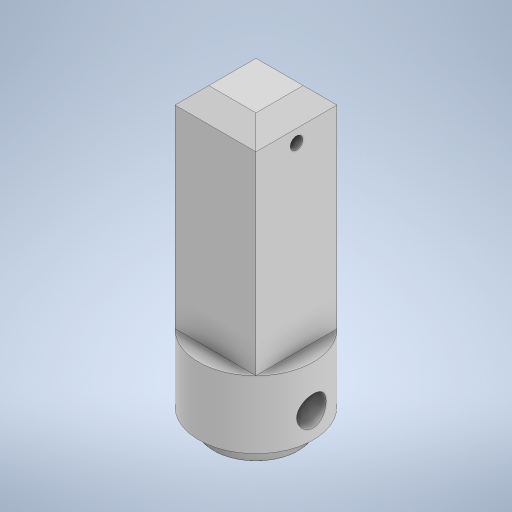
# Autodesk Inventor part: wheel-lockV2
Saved by Autodesk Inventor 2024.2 (Build 282272000, 272)
## iProperties
Created: 2024-04-01
Part Number: wheel-lockV2
Material: Generic
Document SubType Name: Modeling
Designer: Robin
Density: 1 g/cm^3
Appearance: Default
Author: Robin
Autodesk Inventor part; units mm, degrees
ref_plane "YZ Plane" through (0, 0, 0) normal (1, 0, 0) x (0, 1, 0)
ref_plane "XZ Plane" through (0, 0, 0) normal (0, 1, 0) x (-1, 0, 0)
ref_plane "XY Plane" through (0, 0, 0) normal (0, 0, 1) x (1, 0, 0)
sketch "Sketch1" plane through (0, 0, 0) normal (0, 1, 0) x (-1, 0, 0)
  line L0 (4.8, 4.8) -> (-4.8, 4.8)
  line L1 (-4.8, 4.8) -> (-4.8, -4.8)
  line L2 (-4.8, -4.8) -> (4.8, -4.8)
  line L3 (4.8, -4.8) -> (4.8, 4.8)
  point P0 (0, 0)
  point P1 (4.8, 0)
  point P2 (0, -4.8)
  dimension "d0" = 9.6
  dimension "d1" = 9.6
  constraints: 8 end point, 2 midpoint, 2 parallel, 1 horizontal, 1 horizontal alignment, 1 perpendicular, 1 vertical alignment
  measures "d0" distance of L2.end L0.start
  measures "d1" distance of L1.end L2.end
extrude "Extrusion1" add sketch "Sketch1" along normal blind 35
sketch "Sketch5" plane through (0, 0, 0) normal (0, -1, 0) x (1, 0, 0)
  circle A0 centre (0, 0) radius 2.1
  line L0 (4.8, 4.8) -> (4.8, -4.8) projected
  line L1 (-4.8, 4.8) -> (4.8, 4.8) projected
  line L2 (4.8, -4.8) -> (-4.8, -4.8) projected
  line L3 (4.8, 4.8) -> (-4.8, 4.8)
  line L4 (-4.8, 4.8) -> (-4.8, -4.8)
  line L5 (-4.8, -4.8) -> (4.8, -4.8)
  line L6 (4.8, -4.8) -> (4.8, 4.8)
  circle A1 centre (0, 0) radius 6.7882
  point P0 (-4.8, 4.8)
  point P1 (-4.8, 4.8)
  point P2 (-4.8, 4.8)
  dimension "d14" = 4.2
  constraints: 8 end point, 2 coincident, 2 parallel, 1 centre point, 1 horizontal, 1 perpendicular, 3 other
  measures "d14" diameter of A0
extrude "Extrusion5" add sketch "Sketch5" against normal blind 10 contours A1 L0 | L1 A1 | A1 L2 | L4 A1
sketch "Sketch6" plane through (4.8, 35, 4.8) normal (1, 0, 0) x (0, 0, -1)
  line L0 (0, 0) -> (9.6, 0) projected
  point P0 (4.8, -35)
  point P1 (4.8, -3.5)
  point P2 (4.8, 0)
  dimension "d18" = 3.5
  constraints: 1 midpoint, 1 vertical alignment
  measures "d18" distance from line of L0 point (4.8, -3.5)
hole "Hole1" at (4.8, 31.5, 0) direction (-1, 0, 0) diameter 1.5 end through all
sketch "Sketch9" plane through (4.8, 35, 4.8) normal (1, 0, 0) x (0, 0, -1)
  circle A0 centre (4.8, -30) radius 1.75
  point P0 (4.8, -35)
  dimension "d41" = 5
  dimension "d42" = 3.5
  constraints: 1 centre point, 1 vertical alignment
  measures "d41" distance of point (4.8, -35) A0.centre
  measures "d42" diameter of A0
extrude "Extrusion7" cut sketch "Sketch9" along normal blind 5 and the other way blind 4
sketch "Sketch10" plane through (0, 0, 0) normal (0, -1, 0) x (1, 0, 0)
  point P0 (0, 0)
  point P1 (0, 0)
  constraints: 1 coincident
hole "Hole3" at (0, 0, 0) direction (0, 1, 0) diameter 4 depth 9 tip angle 118
sketch "Sketch11" plane through (0, 0, 0) normal (0, -1, 0) x (1, 0, 0)
  circle A0 centre (0, 0) radius 5
  circle A1 centre (0, 0) radius 7.5
  dimension "d55" = 10
  dimension "d63" = 15
  constraints: 2 centre point, 2 coincident
  measures "d55" diameter of A0
  measures "d63" diameter of A1
extrude "Extrusion8" cut sketch "Sketch11" against normal blind 2
fillet "Fillet3" radius 2 1 edges at (-5, 2, 0)
chamfer "Chamfer1" distance 2 angle 45 4 edges at (-4.8, 35, 0) (0, 35, -4.8) (4.8, 35, 0) (0, 35, 4.8)
body "Solid1"
